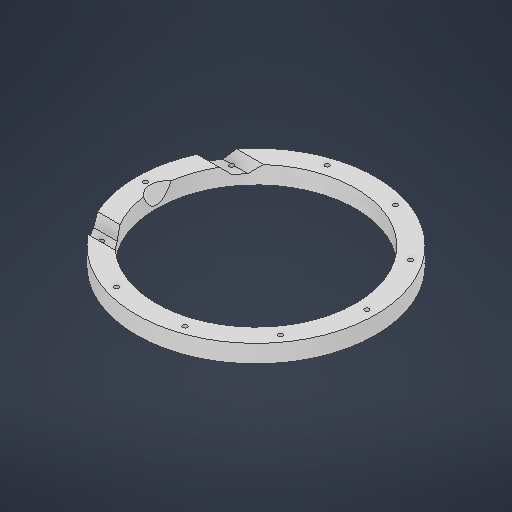
# Autodesk Inventor part: Cylinder Spacer (x3)
Saved by Autodesk Inventor 2025 (Build 290162000, 162)
## iProperties
Created: 2024-04-28
Part Number: Cylinder Spacer (x3)
Material: Generic
Document SubType Name: Modeling
Designer: Thienan Hoang
Density: 1 g/cm^3
Appearance: Default
Author: Thienan Hoang
Autodesk Inventor part; units mm, degrees
ref_plane "YZ Plane" through (0, 0, 0) normal (1, 0, 0) x (0, 1, 0)
sketch "Sketch1" plane through (0, 0, 0) normal (0, 1, 0) x (-1, 0, 0)
  circle A0 centre (0, 0) radius 135
  circle A1 centre (0, 0) radius 112.5
  dimension "d0" = 270
  dimension "d1" = 225
  constraints: 2 centre point, 2 coincident
  measures "d0" diameter of A0
  measures "d1" diameter of A1
extrude "Extrusion1" add sketch "Sketch1" along normal mid plane 20
sketch "Sketch3" plane through (0, 10, 0) normal (0, 1, 0) x (1, 0, 0)
  circle A0 centre (0, 0) radius 125
  circle A1 centre (125, 0) radius 2.5
  circle A2 centre (101.1271, 73.4732) radius 2.5
  circle A3 centre (38.6271, 118.8821) radius 2.5
  circle A4 centre (-38.6271, 118.8821) radius 2.5
  circle A5 centre (-101.1271, 73.4732) radius 2.5
  circle A6 centre (-125, 0) radius 2.5
  circle A7 centre (-101.1271, -73.4732) radius 2.5
  circle A8 centre (-38.6271, -118.8821) radius 2.5
  circle A9 centre (38.6271, -118.8821) radius 2.5
  circle A10 centre (101.1271, -73.4732) radius 2.5
  dimension "d7" = 250
  dimension "d8" = 5
  dimension "d11" = 360
  constraints: 10 centre point, 1 coincident, 1 horizontal alignment, 23 other
  measures "d8" diameter of A1
hole "Hole1" at (125, 10, 0) at (101.1271, 10, 73.4732) at (38.6271, 10, 118.8821) at (-38.6271, 10, 118.8821) at (-101.1271, 10, 73.4732) at (-125, 10, 0) at (-101.1271, 10, -73.4732) at (-38.6271, 10, -118.8821) at (38.6271, 10, -118.8821) at (101.1271, 10, -73.4732) direction (0, -1, 0) diameter 5 end through all
ref_plane "Work Plane6" through (-134.9375, 20, -12.7) normal (0.3947, -0.9188, 0) x (0, 0, 1)
ref_plane "Work Plane7" through (-109.8713, -38.3432, -12.7) normal (0.3947, -0.9188, 0) x (0, 0, 1)
sketch "Sketch5" plane through (-109.8713, -38.3432, -12.7) normal (0.3947, -0.9188, 0) x (0, 0, 1)
  circle A0 centre (12.7, -30.2265) radius 20
  point P0 (12.7, -116.0845)
  dimension "d26" = 40
  dimension "d27" = 85.858
  constraints: 1 centre point
  measures "d26" diameter of A0
  measures "d27" distance of A0.centre point (12.7, -116.085)
extrude "Extrusion4" cut sketch "Sketch5" against normal blind 251.3
sketch "Sketch6" plane through (0, 0, 0) normal (1, 0, 0) x (0, 1, 0)
  line L0 (10, 15.5601) -> (10, -15.5601) projected
  line L1 (10, 0) -> (-10, 0)
  line L2 (-10, -2.5) -> (-10, 2.5) projected
  line L3 (11, -84.799) -> (1.1005, -74.8995)
  line L4 (11, -84.799) -> (25, -84.799) construction
  line L5 (11, -84.799) -> (11, -65)
  line L6 (1.1005, -74.8995) -> (1.1005, -65)
  line L7 (1.1005, -65) -> (11, -55.1005)
  line L8 (1.1005, -65) -> (15.1005, -65) construction
  line L9 (11, -55.1005) -> (11, -65)
  line L10 (11, 84.799) -> (1.1005, 74.8995)
  line L11 (11, 84.799) -> (25, 84.799) construction
  line L12 (11, 84.799) -> (11, 65)
  line L13 (1.1005, 74.8995) -> (1.1005, 65)
  line L14 (1.1005, 65) -> (11, 55.1005)
  line L15 (1.1005, 65) -> (15.1005, 65) construction
  line L16 (11, 55.1005) -> (11, 65)
  point P0 (0, 0)
  dimension "d30" = 14
  dimension "d31" = 135
  dimension "d34" = 65
  dimension "d35" = 14
  dimension "d36" = 45
  constraints: 30 end point, 8 symmetric about line, 2 equal length, 2 horizontal, 2 midpoint, 2 vertical
  measures "d30" distance of L3.start L3.end
  measures "d31" angle of L4 L3
  measures "d34" distance from line of L1 L5.end
  measures "d35" distance of L6.end L7.end
  measures "d36" angle of L8 L7
extrude "Extrusion5" cut sketch "Sketch6" against normal through all
body "Solid1"
